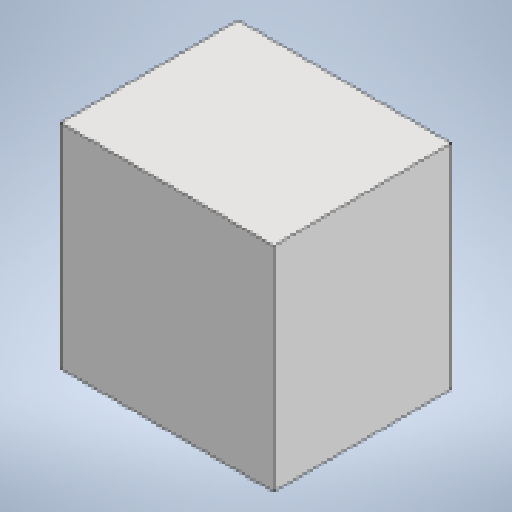
# Autodesk Inventor part: Эскиз рама осн.
Saved by Autodesk Inventor 2025 (Build 290162010, 162A)
## iProperties
Created: 2024-09-30
Part Number: Эскиз рама осн.
Material: Generic
Document SubType Name: Modeling
Designer: pokla
Density: 1 g/cm^3
Appearance: Default
Author: pokla
Autodesk Inventor part; units mm, degrees
ref_plane "YZ Plane" through (0, 0, 0) normal (1, 0, 0) x (0, 1, 0)
ref_plane "XZ Plane" through (0, 0, 0) normal (0, 1, 0) x (-1, 0, 0)
ref_plane "XY Plane" through (0, 0, 0) normal (0, 0, 1) x (1, 0, 0)
sketch "Sketch1" plane through (0, 0, 0) normal (0, 1, 0) x (-1, 0, 0)
  line L0 (960, 960) -> (-960, 960)
  line L1 (-960, 960) -> (-960, -960)
  line L2 (-960, -960) -> (960, -960)
  line L3 (960, -960) -> (960, 960)
  line L4 (960, 960) -> (-960, -960) construction
  point P0 (0, 0)
  point P1 (0, 0)
  dimension "d0" = 1920
  dimension "d1" = 1920
  constraints: 10 end point, 2 parallel, 1 coincident, 1 horizontal, 1 midpoint, 1 perpendicular
  measures "d0" distance of L2.end L0.start
  measures "d1" distance of L0.start L0.end
extrude "Extrusion1" add sketch "Sketch1" along normal blind 1500
body "Solid1"
